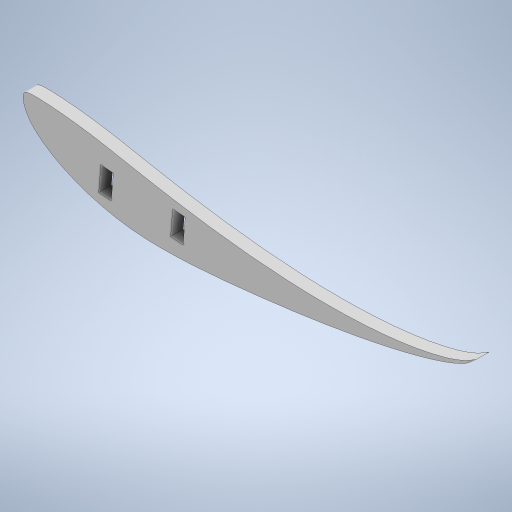
# Autodesk Inventor part: horizontal air foil
Saved by Autodesk Inventor 2024 (Build 280153000, 153)
## iProperties
Created: 2023-07-11
Part Number: horizontal air foil
Material: Generic
Document SubType Name: Modeling
Designer: USER
Density: 1 g/cm^3
Appearance: Default
Author: USER
Autodesk Inventor part; units mm, degrees
ref_plane "YZ Plane" through (0, 0, 0) normal (1, 0, 0) x (0, 1, 0)
ref_plane "XZ Plane" through (0, 0, 0) normal (0, 1, 0) x (-1, 0, 0)
ref_plane "XY Plane" through (0, 0, 0) normal (0, 0, 1) x (1, 0, 0)
sketch "Sketch2" plane through (0, 0, 0) normal (0, 0, 1) x (1, 0, 0)
  spline S0 degree 5 poles (180, 111.4204) (179.9996, 111.416) (179.8254, 111.2846) (179.0647, 110.7171) (178.9747, 110.4647) (177.3489, 109.1041) (176.484, 108.3246) (174.4121, 107.0883) (172.3315, 106.1459) (169.5106, 104.9661) (166.4237, 103.8755) (162.8011, 102.6956) (158.8115, 101.539) (154.3944, 100.354) (149.6145, 99.1823) (144.4796, 98.0168) (139.0304, 96.8737) (133.2934, 95.7516) (127.307, 94.6728) (121.1053, 93.6296) (114.7285, 92.6452) (108.2126, 91.7092) (101.6072, 90.834) (94.9531, 90.0234) (88.3073, 89.2635) (81.719, 88.5836) (75.2467, 87.9844) (68.9286, 87.5133) (62.8071, 87.1758) (56.9035, 87.0433) (51.245, 87.0366) (45.8698, 87.3028) (40.757, 87.8652) (35.8865, 88.646) (31.2785, 89.6753) (26.9182, 90.8702) (22.8356, 92.2269) (19.0417, 93.6976) (15.5573, 95.2911) (12.3953, 96.9641) (9.5692, 98.6998) (7.0968, 100.4855) (4.9719, 102.2705) (3.2341, 104.0734) (1.9141, 105.8904) (0.9025, 107.6678) (0.2861, 109.3358) (-0.0901, 110.9454) (0.0213, 112.3281) (0.2607, 113.7304) (1.7126, 114.1643) (3.555, 114.2426) (5.9608, 114.3253) (8.8453, 114.1531) (12.3003, 113.9413) (16.2663, 113.5524) (20.7439, 113.0545) (25.6739, 112.4187) (31.0535, 111.511) (36.9426, 110.3684) (43.3287, 109.1547) (50.1868, 107.8633) (57.4712, 106.5671) (65.1454, 105.3024) (73.1359, 104.1153) (81.3884, 103.0491) (89.8153, 102.1306) (98.3461, 101.4068) (106.8932, 100.8916) (115.3624, 100.6046) (123.6739, 100.5685) (131.7105, 100.7682) (139.4323, 101.2341) (146.637, 101.8834) (153.4628, 102.8511) (159.3677, 103.7806) (165.134, 105.2605) (169.1123, 106.0961) (173.8338, 108.1363) (175.3383, 108.5113) (178.7035, 110.6488) (178.7146, 110.5539) (179.7873, 111.282) (180.0004, 111.4252) (180, 111.4204) knots 0 0 0 0 0 0 0.00602 0.010963 0.017617 0.025421 0.034068 0.043466 0.053614 0.0645 0.07607 0.08826 0.10101 0.114263 0.127966 0.142066 0.156512 0.171254 0.186243 0.201431 0.216768 0.232202 0.247678 0.263136 0.278514 0.293754 0.308799 0.3236 0.338113 0.352315 0.3662 0.379774 0.393048 0.406034 0.418729 0.431115 0.443167 0.454854 0.466145 0.477009 0.48741 0.497336 0.506781 0.515739 0.524204 0.532169 0.539588 0.546561 0.553486 0.560737 0.568651 0.577556 0.587609 0.59865 0.610538 0.623172 0.636501 0.650486 0.665097 0.680307 0.696073 0.712325 0.728985 0.745973 0.76321 0.780614 0.798102 0.81559 0.83299 0.850213 0.867165 0.88375 0.899867 0.915409 0.930259 0.944279 0.957285 0.969034 0.979253 0.98756 0.993452 1 1 1 1 1 1
  line L0 (180, 96.6734) -> (180, 97.127)
  line L1 (35.8098, 103.3698) -> (34.9992, 93.4027)
  line L2 (34.9992, 93.4027) -> (30.0156, 93.8081)
  line L3 (30.0156, 93.8081) -> (30.8263, 103.7751)
  line L4 (30.8263, 103.7751) -> (35.8098, 103.3698)
  line L5 (64.3505, 102.4875) -> (63.5398, 92.5204)
  line L6 (63.5398, 92.5204) -> (58.5563, 92.9258)
  line L7 (58.5563, 92.9258) -> (59.367, 102.8929)
  line L8 (59.367, 102.8929) -> (64.3505, 102.4875)
  point P0 (178.9506, 110.5312)
  point P1 (177.885, 109.5538)
  point P2 (176.535, 108.4576)
  point P3 (174.7998, 107.3704)
  point P4 (172.5912, 106.285)
  point P5 (169.9002, 105.1636)
  point P6 (166.7502, 104.0116)
  point P7 (163.1538, 102.838)
  point P8 (159.1308, 101.6518)
  point P9 (154.7046, 100.4602)
  point P10 (149.8986, 99.2722)
  point P11 (144.7416, 98.0968)
  point P12 (139.2642, 96.9412)
  point P13 (133.4988, 95.8126)
  point P14 (127.4814, 94.7218)
  point P15 (121.248, 93.6742)
  point P16 (114.8364, 92.6788)
  point P17 (108.2844, 91.7374)
  point P18 (101.637, 90.8554)
  point P19 (94.9392, 90.0346)
  point P20 (88.245, 89.275)
  point P21 (81.612, 88.591)
  point P22 (75.0978, 88.0006)
  point P23 (68.7474, 87.5326)
  point P24 (62.5986, 87.2158)
  point P25 (56.6784, 87.0736)
  point P26 (51.0246, 87.1114)
  point P27 (45.666, 87.3976)
  point P28 (40.5738, 87.9538)
  point P29 (35.7228, 88.7512)
  point P30 (31.1148, 89.7736)
  point P31 (26.7534, 90.9814)
  point P32 (22.6638, 92.344)
  point P33 (18.8676, 93.8344)
  point P34 (15.381, 95.4382)
  point P35 (12.2202, 97.1284)
  point P36 (9.4014, 98.8834)
  point P37 (6.939, 100.678)
  point P38 (4.8492, 102.4816)
  point P39 (3.159, 104.2906)
  point P40 (1.8504, 106.1032)
  point P41 (0.891, 107.8762)
  point P42 (0.279, 109.561)
  point P43 (0.009, 111.1)
  point P44 (0.0792, 112.4302)
  point P45 (0.4752, 113.4364)
  point P46 (1.4202, 113.989)
  point P47 (3.0924, 114.2104)
  point P48 (5.4108, 114.2716)
  point P49 (8.3286, 114.178)
  point P50 (11.8098, 113.9476)
  point P51 (15.8166, 113.584)
  point P52 (20.3076, 113.0854)
  point P53 (25.236, 112.4338)
  point P54 (30.6108, 111.5554)
  point P55 (36.5004, 110.4574)
  point P56 (42.912, 109.237)
  point P57 (49.8114, 107.95)
  point P58 (57.15, 106.6468)
  point P59 (64.8792, 105.376)
  point P60 (72.9342, 104.1826)
  point P61 (81.2502, 103.108)
  point P62 (89.748, 102.1882)
  point P63 (98.3502, 101.4592)
  point P64 (106.9704, 100.9444)
  point P65 (115.5168, 100.6636)
  point P66 (123.8976, 100.6312)
  point P67 (132.0192, 100.8508)
  point P68 (139.788, 101.3188)
  point P69 (147.1122, 102.0262)
  point P70 (153.9, 102.9496)
  point P71 (160.0704, 104.062)
  point P72 (165.5388, 105.3238)
  point P73 (170.2314, 106.6972)
  point P74 (174.0474, 108.1408)
  point P75 (176.859, 109.5124)
  point P76 (178.6824, 110.578)
  point P77 (179.685, 111.2134)
  point P78 (95.0285, 99.5434)
  constraints: 18 end point, 80 other
extrude "Extrusion1" add sketch "Sketch2" along normal blind 5
body "Solid1"
